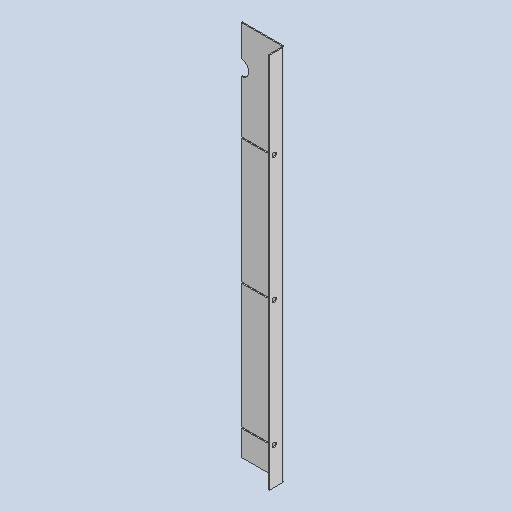
# Autodesk Inventor part: GBK 0104 stringer 3
Saved by Autodesk Inventor 2026.2 (Build 302298000, 298)
## iProperties
Manager: 28
Created: 2026-05-07
Part Number: GBK 0104 stringer 3
Material: Steel
Document SubType Name: Sheet Metal
Designer: pokla
Density: 7.85 g/cm^3
Sheet Metal Rule: Default_mm
Appearance: Default
Mass: 10239.7 g
Surface Area: 6691.22 cm^2
Volume: 1304.42 cm^3
Flat Pattern Width: 22.1067 cm
Flat Pattern Length: 148.95 cm
Flat Pattern Area: 3292.79 cm^2
Sheet Metal Width: 221,067 mm
Sheet Metal Length: 1489,500 mm
Sheet Metal Area: 329278,961 mm^2
Stock Number: 0104
Description: 28
Author: admin
Revision Number: 28
Autodesk Inventor part; units mm, degrees
ref_plane "YZ Plane" through (0, 0, 0) normal (1, 0, 0) x (0, 1, 0)
ref_plane "XZ Plane" through (0, 0, 0) normal (0, 1, 0) x (-1, 0, 0)
ref_plane "XY Plane" through (0, 0, 0) normal (0, 0, 1) x (1, 0, 0)
sketch "Sketch1" plane through (0, 0, 0) normal (0, 0, 1) x (1, 0, 0)
  line L0 (0, 0) -> (-168.019, 0)
  line L1 (-168.019, 0) -> (-168.019, -1489.5)
  line L2 (-168.019, -1489.5) -> (0, -1489.5)
  line L3 (0, -1489.5) -> (0, 0)
  line L4 (-168.019, -1389.5) -> (-66, -1389.5)
  line L5 (-66, -1389.5) -> (-66, -1384.5)
  line L6 (-66, -1384.5) -> (-168.019, -1384.5)
  line L7 (-168.019, -1384.5) -> (-168.019, -1389.5)
  line L8 (-168.019, -892.8333) -> (-66, -892.8333)
  line L9 (-66, -892.8333) -> (-66, -887.8333)
  line L10 (-66, -887.8333) -> (-168.019, -887.8333)
  line L11 (-168.019, -887.8333) -> (-168.019, -892.8333)
  line L12 (-168.019, -396.1667) -> (-66, -396.1667)
  line L13 (-66, -396.1667) -> (-66, -391.1667)
  line L14 (-66, -391.1667) -> (-168.019, -391.1667)
  line L15 (-168.019, -391.1667) -> (-168.019, -396.1667)
  circle A0 centre (-168.019, -154.5) radius 30
  point P0 (-168.019, -396.1667)
  point P1 (-168.019, -124.5)
  point P2 (-168.019, -184.5)
  dimension "d0" = 1489.5
  dimension "d1" = 168.019
  dimension "d2" = 5
  dimension "d4" = 100
  dimension "d7" = 496.6667
  dimension "d23" = 66
  dimension "d28" = 60
  dimension "d29" = 1335
  measures "d0" distance of L1.end L0.end
  measures "d1" distance of L1.end L2.end
  measures "d2" distance of L4.end L5.end
  measures "d4" distance between parallel lines of L2 L4
  measures "d7" distance of L4.start L8.start
  measures "d23" distance between parallel lines of L3 L5
  measures "d28" diameter of A0
  measures "d29" distance from line of A0.centre L2
extrude "Plate1" add sketch "Sketch1" along normal blind 4 contours L3 L2 L1 L4 L5 L6 L8 L9 L10 L12 L13 L14 A0 L0
sketch "Sketch2" plane through (-4, 0, 0) normal (1, 0, 0) x (0, 1, 0)
  line L0 (-1489.5, 0) -> (0, 0)
  line L1 (0, 0) -> (0, 60)
  line L2 (0, 60) -> (-1489.5, 60)
  line L3 (-1489.5, 60) -> (-1489.5, 0)
  constraints: 6 end point, 1 horizontal, 1 perpendicular, 1 vertical
edge flange "Flange1" height 60 angle 90 thickness 4 bend radius 4 thickness toward (1, 0, 0) relief straight relief width 4 relief depth 2 edges at (0, -744.75, 4) wall of the first edge with corners at (-4, -1489.5, 0) (-4, 0, 0) (-4, 0, 60) (-4, -1489.5, 60)
bend "Bend1"
corner "Corner1"
chamfer "Corner Chamfer1" distance 3 angle 45 6 edges at (-168.019, -1389.5, 2) (-168.019, -1384.5, 2) (-168.019, -892.8333, 2) (-168.019, -887.8333, 2) (-168.019, -391.1667, 2) (-168.019, -396.1667, 2)
sketch "Sketch4" plane through (0, -1489.5, 60) normal (1, 0, 0) x (0, 0, -1)
  line L0 (52, 0) -> (52, 1489.5) construction
  line L1 (0, 1489.5) -> (52, 1489.5) construction
  line L2 (0, 0) -> (0, 1489.5) construction
  line L3 (52, 0) -> (0, 0) construction
  circle A0 centre (18, 1139.5) radius 9
  circle A1 centre (18, 642.8333) radius 9
  circle A2 centre (18, 146.1667) radius 9
  point P0 (60, 1489.5)
  dimension "d30" = 18
  dimension "d31" = 18
  dimension "d32" = 350
  dimension "d35" = 496.6667
  constraints: 3 centre point, 1 vertical, 4 other
  measures "d30" diameter of A0
  measures "d31" distance from line of L2 A0.centre
  measures "d32" distance from line of A0.centre L1
  measures "d35" distance of A0.centre A1.centre
extrude "Cut1" cut sketch "Sketch4" against normal blind 4
equation "\"d0\" = Стрингер_длина"
equation "\"d1\" = стрингер_глубина_3"
equation "\"d2\" = паз_под_стрингер_толщина"
equation "\"d7\" = Шаг_шпангоутов"
equation "\"d23\" = паз_под_стрингер_глубина - Thickness"
equation "\"d28\" = 2 * радиус_выреза_под_сварку"
equation "\"d35\" = Шаг_шпангоутов"
equation "\"d40\" = Thickness"
equation "\"d12\" = Thickness"
equation "\"d13\" = BendReliefWidth"
equation "\"d14\" = BendReliefDepth"
equation "\"d15\" = MinimumRemnant"
equation "\"d16\" = TransitionRadius"
equation "\"d17\" = ребро_усилителей"
equation "\"d19\" = BendRadius"
equation "\"d20\" = CornerReliefSize"
equation "\"d21\" = GapSize"
equation "\"d22\" = JacobiRadiusSize"
equation "\"BendRadius\" = Thickness"
equation "\"BendReliefWidth\" = Thickness"
equation "\"BendReliefDepth\" = 0.5 * Thickness"
equation "\"CornerReliefSize\" = 4 * Thickness"
equation "\"MinimumRemnant\" = 2 * Thickness"
equation "\"TransitionRadius\" = BendRadius"
equation "\"JacobiRadiusSize\" = BendRadius"
equation "\"GapSize\" = Thickness"
equation "\"Стрингер_длина\" = 1489.5"
equation "\"стрингер_глубина_3\" = 168.018988"
equation "\"паз_под_стрингер_толщина\" = 5"
equation "\"Шаг_шпангоутов\" = 496.666667"
equation "\"паз_под_стрингер_глубина\" = 70"
equation "\"Thickness\" = 4"
equation "\"радиус_выреза_под_сварку\" = 30"
equation "\"ребро_усилителей\" = 60"
body "Solid1"
